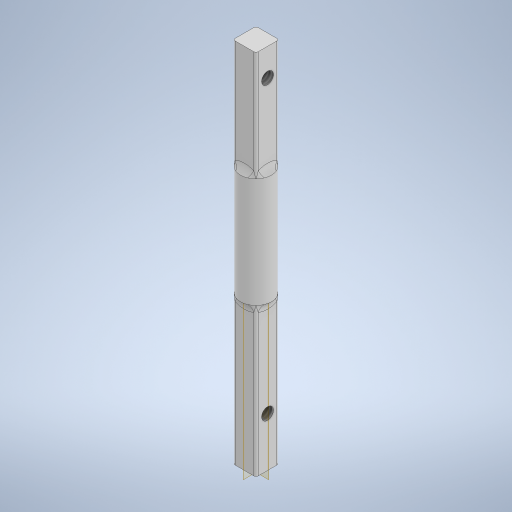
# Autodesk Inventor part: DrivenShaft
Saved by Autodesk Inventor 2023.2 (Build 272271030, 271C)
## iProperties
Created: 2023-02-19
Part Number: DrivenShaft
Material: Generic
Document SubType Name: Modeling
Designer: atrus
Density: 1 g/cm^3
Appearance: Default
Author: atrus
Autodesk Inventor part; units mm, degrees
ref_plane "YZ Plane" through (0, 0, 0) normal (1, 0, 0) x (0, 1, 0)
ref_plane "XZ Plane" through (0, 0, 0) normal (0, 1, 0) x (-1, 0, 0)
ref_plane "XY Plane" through (0, 0, 0) normal (0, 0, 1) x (1, 0, 0)
sketch "Sketch1" plane through (0, 0, 0) normal (0, 1, 0) x (-1, 0, 0)
  line L0 (4.207285, 0) -> (0, 0)
  line L1 (0, 0) -> (0, -4.207285)
  line L2 (0, -4.207285) -> (4.207285, -4.207285)
  line L3 (4.207285, -4.207285) -> (4.207285, 0)
  dimension "d0" = 5.95
  constraints: 8 end point, 2 parallel, 2 perpendicular, 1 coincident, 1 horizontal
  measures "d0" distance of L1.end L0.start
extrude "Extrusion1" add sketch "Sketch1" along normal blind 27
sketch "Sketch2" plane through (0, 0, 0) normal (1, 0, 0) x (0, 0, -1)
  line L0 (0, 0) -> (4.207285, 0) construction
  line L1 (0, 27) -> (4.207285, 27) construction
  line L2 (2.103643, 0) -> (2.103643, 27) construction
  point P0 (2.103643, 9)
  dimension "d3" = 9
  constraints: 2 end point, 2 midpoint, 1 point on line
  measures "d3" distance from line of L0 point (2.104, 9)
hole "Hole1" at (0, 9, -2.103643) direction (-1, 0, 0) diameter 2.15646 end through all thread size "4-40 UNC" class "2B" standard "ANSI Unified Screw Threads"
fillet "Fillet1" radius 0.4 4 edges at (-4.2073, 13.5, 0) (-4.2073, 13.5, -4.2073) (0, 13.5, -4.2073) (0, 13.5, 0)
ref_plane "Work Plane1" through (-2.103643, 0, -0.4) normal (1, 0, 0) x (0, 0, -1)
ref_plane "Work Plane2" through (-3.807285, 0, -2.103643) normal (0, 0, 1) x (1, 0, 0)
sketch "Sketch3" plane through (0, 27, 0) normal (0, 1, 0) x (1, 0, 0)
  arc A0 (-0.4, 0) -> (0, 0.4) centre (-0.4, 0.4) ccw construction
  line L0 (0, 0.4) -> (0, 3.807285) construction
  arc A1 (0, 3.807285) -> (-0.4, 4.207285) centre (-0.4, 3.807285) ccw construction
  line L1 (-0.4, 4.207285) -> (-3.807285, 4.207285) construction
  arc A2 (-3.807285, 4.207285) -> (-4.207285, 3.807285) centre (-3.807285, 3.807285) ccw construction
  line L2 (-4.207285, 3.807285) -> (-4.207285, 0.4) construction
  arc A3 (-4.207285, 0.4) -> (-3.807285, 0) centre (-3.807285, 0.4) ccw construction
  line L3 (-3.807285, 0) -> (-0.4, 0) construction
  circle A4 centre (-2.103643, 2.103643) radius 2.809315
  point P0 (0, 0)
  constraints: 1 centre point
extrude "Extrusion2" add sketch "Sketch3" along normal blind 20
sketch "Sketch4" plane through (-2.103643, 47, -2.103643) normal (0, 1, 0) x (1, 0, 0)
  arc A0 (1.703643, -2.103643) -> (2.103643, -1.703643) centre (1.703643, -1.703643) ccw
  line L0 (-1.703643, -2.103643) -> (1.703643, -2.103643)
  arc A1 (-2.103643, -1.703643) -> (-1.703643, -2.103643) centre (-1.703643, -1.703643) ccw
  line L1 (-2.103643, 1.703643) -> (-2.103643, -1.703643)
  arc A2 (-1.703643, 2.103643) -> (-2.103643, 1.703643) centre (-1.703643, 1.703643) ccw
  line L2 (1.703643, 2.103643) -> (-1.703643, 2.103643)
  arc A3 (2.103643, 1.703643) -> (1.703643, 2.103643) centre (1.703643, 1.703643) ccw
  line L3 (2.103643, -1.703643) -> (2.103643, 1.703643)
  point P0 (2.103643, -2.103643)
extrude "Extrusion3" add sketch "Sketch4" along normal blind 20
sketch "Sketch6" plane through (-4.207285, 47, -3.807285) normal (-1, 0, 0) x (0, 0, 1)
  line L0 (3.407285, 20) -> (0, 20) construction
  line L1 (1.703643, 20) -> (1.703643, 0) construction
  line L2 (0, 0) -> (3.407285, 0) construction
  point P0 (3.807285, -47)
  point P1 (1.703643, 15)
  dimension "d23" = 5
  constraints: 2 end point, 2 midpoint, 1 point on line
  measures "d23" distance from line of L0 point (1.704, 15)
hole "Hole3" at (-4.207285, 62, -2.103643) direction (1, 0, 0) diameter 2.15646 depth 8.865 tip angle 118 thread size "4-40 UNC" class "2B" standard "ANSI Unified Screw Threads"
fillet "Fillet2" radius 2 24 edges at (-4.1768, 47, -3.9604) (-4.1768, 47, -0.2469) (-4.2073, 47, -2.1036) (-0.2469, 47, -4.1768) (-3.9604, 47, -4.1768) (-2.1036, 47, -4.2073) (-3.9604, 47, -0.0304) (-0.2469, 47, -0.0304) (-2.1036, 47, 0) (-0.0304, 47, -0.2469) (-0.0304, 47, -3.9604) (0, 47, -2.1036) (-0.2469, 27, -0.0304) (-3.9604, 27, -0.0304) (-2.1036, 27, 0) (-0.0304, 27, -3.9604) (-0.0304, 27, -0.2469) (0, 27, -2.1036) (-4.1768, 27, -0.2469) (-4.1768, 27, -3.9604) (-4.2073, 27, -2.1036) (-3.9604, 27, -4.1768) (-0.2469, 27, -4.1768) (-2.1036, 27, -4.2073)
body "Solid1"
